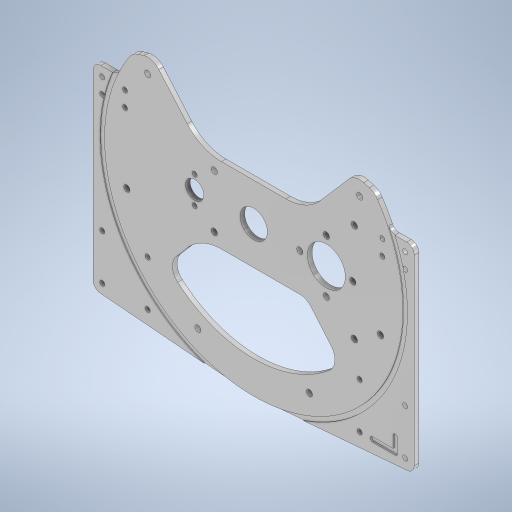
# Autodesk Inventor part: TH22_motorboard_775_v3
Saved by Autodesk Inventor 2024.1 (Build 281209000, 209)
## iProperties
Created: 2021-11-15
Part Number: TH22_motorboard_775_v3
Material: アルミニウム 6061-AHC
Document SubType Name: Modeling
Designer: 中島 青蔵
Density: 2.7 g/cm^3
Appearance: アルミニウム - ダーク
Author: 中島 青蔵
Autodesk Inventor part; units mm, degrees
ref_plane "YZ Plane" through (0, 0, 0) normal (1, 0, 0) x (0, 1, 0)
ref_plane "XZ Plane" through (0, 0, 0) normal (0, 1, 0) x (-1, 0, 0)
ref_plane "XY Plane" through (0, 0, 0) normal (0, 0, 1) x (1, 0, 0)
sketch "スケッチ1" plane through (0, 0, 0) normal (0, 0, 1) x (1, 0, 0)
  circle A0 centre (0, 0) radius 9
  line L0 (-50, 25) -> (50, 25)
  line L1 (50, 25) -> (50, -25)
  line L2 (50, -25) -> (-50, -25)
  line L3 (-50, -25) -> (-50, 25)
  line L4 (-15.8002, 25) -> (-50, 7.5852)
  line L5 (0, 0) -> (0, 25)
  line L6 (-50, 0) -> (0, 0)
  line L7 (15.8002, 25) -> (50, 7.5852)
  line L8 (20.5424, -25) -> (50, -10)
  circle A1 centre (0, 0) radius 77
  line L9 (50, 7.5852) -> (79.5557, 42.8084)
  line L10 (50, 7.5852) -> (95.9806, 7.5852) construction
  line L11 (35, 25) -> (62.1783, 57.3898)
  line L12 (35, 25) -> (77.2819, 25) construction
  line L13 (62.1783, 57.3898) -> (79.5557, 42.8084)
  line L14 (-50, 0) -> (50, 0)
  line L15 (50, -10) -> (79.5557, -42.8084)
  line L16 (35, -25) -> (62.1783, -57.3898)
  line L17 (62.1783, -57.3898) -> (79.5557, -42.8084)
  line L18 (-50, 7.5852) -> (-79.5557, 42.8084)
  line L19 (-35, 25) -> (-62.1783, 57.3898)
  line L20 (-62.1783, 57.3898) -> (-79.5557, 42.8084)
  line L21 (-35, -25) -> (-62.1783, -57.3898)
  line L22 (-50, -10) -> (-79.5557, -42.8084)
  line L23 (-62.1783, -57.3898) -> (-79.5557, -42.8084)
  line L24 (0, 0) -> (62.2943, 45.2595)
  line L25 (0, 0) -> (74.5809, -19.1491)
  line L26 (0, 0) -> (32.785, -69.6717)
  line L27 (0, 0) -> (-62.2943, 45.2595)
  line L28 (0, 0) -> (-74.5809, -19.1491)
  line L29 (0, 0) -> (-32.785, -69.6717)
  circle A2 centre (69.98, 50.8434) radius 9.5
  circle A3 centre (69.98, 50.8434) radius 2
  circle A4 centre (0, 0) radius 86.5
  circle A5 centre (83.7824, -21.5117) radius 2
  circle A6 centre (36.8299, -78.2675) radius 2
  circle A7 centre (69.98, 50.8434) radius 5
  circle A8 centre (83.7824, -21.5117) radius 5
  circle A9 centre (36.8299, -78.2675) radius 5
  circle A10 centre (-69.98, 50.8434) radius 2
  circle A11 centre (-83.7824, -21.5117) radius 2
  circle A12 centre (-36.8299, -78.2675) radius 2
  circle A13 centre (-69.98, 50.8434) radius 5
  circle A14 centre (-83.7824, -21.5117) radius 5
  circle A15 centre (-36.8299, -78.2675) radius 5
  circle A16 centre (0, 0) radius 98.5
  circle A17 centre (-69.98, 50.8434) radius 9.5
  line L30 (-74.3377, 60.3434) -> (117.0207, 60.3434)
  line L31 (-35, 25) -> (-62.8021, 57.0667)
  line L32 (35, 25) -> (62.8021, 57.0667)
  line L33 (-62.2943, 45.2595) -> (-79.6882, 57.8968)
  line L34 (-79.6882, 57.8968) -> (-72.6529, 59.9596)
  line L35 (79.6882, 57.8968) -> (72.6529, 59.9596)
  circle A18 centre (48, 0) radius 24
  circle A19 centre (-39, 0) radius 6
  circle A20 centre (-39, 9) radius 1.6
  circle A21 centre (-39, -9) radius 1.6
  circle A22 centre (0, 0) radius 24
  circle A23 centre (-39, 0) radius 15
  point P0 (50, 7.5852)
  point P1 (49.9991, -10)
  point P2 (50, -10)
  point P3 (50, 7.5852)
  point P4 (15.8002, 25)
  point P5 (50.0002, -9.8901)
  point P6 (-50.0002, -10)
  point P7 (62.2943, 45.2595)
  point P8 (57.2394, 51.5039)
  point P9 (70.1939, 31.6514)
  point P10 (69.9626, -32.1595)
  point P11 (57.2394, -51.5039)
  point P12 (-57.2394, -51.5039)
  point P13 (-69.9626, -32.1595)
  point P14 (-70.1939, 31.6514)
  point P15 (-57.2394, 51.5039)
  point P16 (-77.6656, 56.4274)
  point P17 (77.6656, 56.4274)
  point P18 (-62.7025, 56.9499)
  point P19 (62.7025, 56.9499)
  point P20 (-62.7016, 56.9507)
  point P21 (62.7016, 56.9507)
  point P22 (53.3257, -13.6917)
  point P23 (46.2951, -11.8866)
  point P24 (11.7641, -25)
  dimension "d78" = 197
  dimension "d0" = 18
  dimension "d7" = 50
  dimension "d27" = 100
  dimension "d43" = 154
  dimension "d44" = 50
  dimension "d45" = 50
  dimension "d58" = 25
  dimension "d59" = 15
  dimension "d63" = 15
  dimension "d67" = 15
  dimension "d68" = 54
  dimension "d69" = 50.4
  dimension "d70" = 50.4
  dimension "d71" = 19
  dimension "d72" = 4
  dimension "d73" = 4
  dimension "d74" = 4
  dimension "d75" = 10
  dimension "d76" = 10
  dimension "d77" = 10
  dimension "d118" = 48
  dimension "d119" = 48
  dimension "d172" = 12
  dimension "d173" = 3.2
  dimension "d174" = 3.2
  dimension "d175" = 9
  dimension "d176" = 9
  dimension "d177" = 48
  dimension "d178" = 30
  dimension "d179" = 0
  dimension "d180" = 0
  constraints: 72 end point, 26 symmetric about line, 23 centre point, 14 coincident, 9 point on line, 8 point on circle, 6 tangent, 3 midpoint, 3 perpendicular, 2 equal length, 2 horizontal, 1 collinear, 1 parallel, 1 vertical, 10 other
  measures "d0" diameter of A0
  measures "d7" distance of L0.end L1.end
  measures "d27" distance of L0.start L0.end
  measures "d43" diameter of A1
  measures "d44" angle of L10 L9
  measures "d45" angle of L12 L11
  measures "d58" distance from line of point (0, 0) L2
  measures "d59" distance from line of L2 L8.end
  measures "d63" distance of L0.end L11.start
  measures "d67" distance of L2.end point (-50, -10)
  measures "d68" angle of L5 L24
  measures "d69" angle of L24 L25
  measures "d70" angle of L25 L26
  measures "d71" diameter of A2
  measures "d72" diameter of A3
  measures "d73" diameter of A5
  measures "d74" diameter of A6
  measures "d75" diameter of A7
  measures "d76" diameter of A8
  measures "d77" diameter of A9
  measures "d118" distance of point (0, 0) point (48, 0)
  measures "d119" diameter of A18
  measures "d172" diameter of A19
  measures "d173" diameter of A20
  measures "d174" diameter of A21
  measures "d175" distance of A19.centre A20.centre
  measures "d176" distance of A21.centre A19.centre
  measures "d177" diameter of A22
  measures "d178" diameter of A23
  measures "d179" horizontal distance of A19.centre A20.centre
  measures "d180" horizontal distance of A19.centre A21.centre
extrude "押し出し1" add sketch "スケッチ1" along normal blind 3 contours L14 A22 L25 A0 | A0 L24 A22 L14 | A0 L5 A22 L24 | L25 A22 L26 A0 | A18 L7 L1 L14 | A22 L24 L7 A18 | L14 L1 L8 L25 A18 | A18 L25 A22 | A0 L27 A22 L5 | A22 L5 L0 L7 L24 | L26 A22 L29 A0 | L25 A18 L8 L2 L26 A22 | L6 A22 L27 A0 | A0 L28 A22 L6 | A0 L29 A22 L28 | L1 L9 A18 L25 L15 | A18 L1 L7 | L7 L24 L0 L1 A18 | L25 L8 A18 | A22 L27 L4 L0 L5 | L7 L0 L24 | L26 L2 L29 A22 | A23 L28 A21 L3 L6 A19 | A23 L4 L27 A22 | L6 A19 L3 L4 A23 | A22 L28 A23 | A22 L29 L2 L3 L28 A23 | L1 A18 L9 | L15 L25 L1 | L1 L25 L8 | L1 L0 L32 L24 A1 L9 A18 | L25 L1 A18 L8 | A18 L1 L2 L8 | A23 L3 L0 L27 L4 | L4 L3 A23 | A23 L28 A21 | L27 L0 L4 | L9 A1 L25 A18 | L25 L15 A18 L1 | L25 A18 L15 | A18 L15 A1 L16 L2 L1 | A1 L16 L17 A4 A9 A15 L23 L21 | L18 A23 L3 | L3 L22 A23 L18 | A23 L18 A1 L27 L31 L0 L3 | L28 L3 A23 | L21 A1 L22 L28 L3 L2 | L9 A4 A8 L15 A1 | A1 A2 A4 L9 | A18 L25 A1 L15 | L32 A1 L24 | A1 L15 A4 L17 L16 | A23 L22 L28 A1 L18 | L28 L22 A23 L3 | A23 L22 L3 | L21 L23 A4 L22 A1 | A1 L32 A2 | A2 L13 A7 A4 | A4 A2 L13 L9 | L9 L13 A2 L35 A16 L33 A17 L20 L18 A4 A14 L22 L23 A15 A9 L17 L15 A8 | L18 A4 A17 A1 | A1 L22 A4 A14 L18 | L22 A1 L28 | L27 A1 L31 | A2 A4 A7 L13 | A4 A7 L13 A2 | L15 L17 A4 | A17 L31 A1 | L33 A13 L20 A17 | A17 A4 A13 L33 | L18 L20 A17 A4 | A4 L23 L22 | A7 A4 A3 L13 | L13 A3 A4 A7 | L13 A7 A4 A2 | A4 A3 L13 A7 | A8 A4 A5 | A4 A5 A8 | A9 A4 A6 | A4 A6 A9 | A17 L20 A13 A4 | L33 A10 L20 A13 | A13 A4 A10 L33 | A14 A4 A11 | A4 A11 A14 | L20 A13 A4 A17 | A15 A4 A12 | A4 A12 A15 | A7 L13 A3 A4 | A4 A13 L33 A17 | A13 L20 A10 A4 | A17 L33 A13 L20 | L20 A10 A4 A13 | A4 A10 L33 A13 | A17 L33 L34 | A13 L33 A10 L20
fillet "フィレット2" radius 30 3 edges at (35, 25, 1.5) (-35, -25, 1.5) (-35, 25, 1.5)
fillet "フィレット5" radius 10 5 edges at (-79.6882, 57.8968, 1.5) (79.6882, 57.8968, 1.5) (-57.2394, -51.5039, 1.5) (35, -25, 1.5) (57.2394, -51.5039, 1.5)
sketch "スケッチ6" plane through (0, 0, 3) normal (0, 0, 1) x (1, 0, 0)
  point P0 (0, 0)
  point P1 (48, 0)
  point P2 (48, 17.5)
  point P3 (30.5, 0)
  point P4 (48, -17.5)
  point P5 (65.5, 0)
  dimension "d81" = 48
  dimension "d82" = 17.5
  dimension "d85" = 360
  constraints: 5 other
  measures "d81" distance of point (0, 0) point (48, 0)
  measures "d82" distance of point (48, 0) point (48, 17.5)
hole "穴4" at (48, 0, 3) direction (0, 0, -1) diameter 25 depth 8 tip angle 118
hole "穴5" at (48, 17.5, 3) at (30.5, 0, 3) at (48, -17.5, 3) at (65.5, 0, 3) direction (0, 0, -1) diameter 4 depth 8 tip angle 118
sketch "スケッチ7" plane through (0, 0, 3) normal (0, 0, 1) x (1, 0, 0)
  line L0 (21.3047, 25) -> (-21.3047, 25) projected
  line L1 (-21.0108, -25) -> (30.3369, -25) projected
  circle A0 centre (48, 0) radius 12.5 projected
  point P0 (0, 0)
  point P1 (-26, 17.5)
  point P2 (-26, -17.5)
  point P3 (66.5, -32.5)
  point P4 (66.5, 32.5)
  point P5 (21.0108, -25)
  point P6 (11.7641, -25)
  point P7 (5.4179, -25)
  point P8 (25.7007, -25)
  point P9 (-35, -25)
  point P10 (35, -25)
  point P11 (-30.3369, -25)
  dimension "d101" = 26
  dimension "d102" = 7.5
  dimension "d103" = 26
  dimension "d104" = 7.5
  dimension "d105" = 18.5
  dimension "d106" = 18.5
  dimension "d116" = 7.5
  dimension "d117" = 7.5
  constraints: 1 other
  measures "d101" horizontal distance of point (0, 0) point (-26, 17.5)
  measures "d102" distance from line of L0 point (-26, 17.5)
  measures "d103" horizontal distance of point (-26, -17.5) point (0, 0)
  measures "d105" horizontal distance of A0.centre point (66.5, 32.5)
  measures "d106" horizontal distance of A0.centre point (66.5, -32.5)
  measures "d116" distance from line of L0 point (66.5, 32.5)
hole "穴6" at (-26, 17.5, 3) at (-26, -17.5, 3) at (66.5, -32.5, 3) at (66.5, 32.5, 3) direction (0, 0, -1) diameter 4 depth 8 tip angle 118
sketch "スケッチ8" plane through (0, 0, 3) normal (0, 0, 1) x (1, 0, 0)
  arc A0 (-81.8095, 54.8585) -> (81.8095, 54.8585) centre (0, 0) ccw projected
  circle A1 centre (83.7824, -21.5117) radius 2 projected
  line L0 (89.9517, 40.1366) -> (106, 40.1366)
  line L1 (106, 40.1366) -> (106, -89.8634)
  line L2 (106, -89.8634) -> (8.3243, -98.1476)
  line L3 (0, 0) -> (0, -98.5)
  circle A2 centre (100, 34.1366) radius 1.6
  circle A3 centre (100, -83.8634) radius 1.6
  line L4 (-89.9517, 40.1366) -> (-106, 40.1366)
  line L5 (-106, 40.1366) -> (-106, -89.8634)
  line L6 (-106, -89.8634) -> (-8.3243, -98.1476)
  circle A4 centre (-100, 34.1366) radius 1.6
  circle A5 centre (-100, -83.8634) radius 1.6
  point P0 (-8.3243, -98.1476)
  point P1 (-89.9517, 40.1366)
  dimension "d132" = 130
  dimension "d133" = 3.2
  dimension "d134" = 3.2
  dimension "d135" = 6
  dimension "d136" = 6
  dimension "d137" = 6
  dimension "d138" = 6
  dimension "d155" = 85.152
  dimension "d156" = 100
  constraints: 14 end point, 6 symmetric about line, 4 centre point, 3 point on circle, 1 horizontal, 1 tangent, 1 vertical, 2 other
  measures "d132" distance of L0.end L1.end
  measures "d133" diameter of A2
  measures "d134" diameter of A3
  measures "d135" distance from line of L0 A2.centre
  measures "d136" distance from line of L1 A2.centre
  measures "d137" distance from line of L1 A3.centre
  measures "d138" horizontal distance of L1.end A3.centre
  measures "d155" angle of L3 L2
  measures "d156" horizontal distance of point (0, 0) A2.centre
extrude "押し出し2" add sketch "スケッチ8" against normal blind 3 contours A0 L6 L5 L4 | A0 L0 L1 L2
fillet "フィレット8" radius 5 6 edges at (106, 40.1366, 1.5) (106, -89.8634, 1.5) (-106, -89.8634, 1.5) (-106, 40.1366, 1.5) (-89.9517, 40.1366, 1.5) (89.9517, 40.1366, 1.5)
sketch "スケッチ9" plane through (0, 0, 3) normal (0, 0, 1) x (1, 0, 0)
  arc A0 (-81.8095, 54.8585) -> (81.8095, 54.8585) centre (0, 0) ccw projected
  circle A1 centre (0, 0) radius 101.5
  arc A2 (88.6399, 42.9561) -> (93.1393, 40.1366) centre (93.1393, 45.1366) ccw projected
  line L0 (8.3243, -98.1476) -> (101.4226, -90.2516) projected
  line L1 (-101.4226, -90.2516) -> (-8.3243, -98.1476) projected
  arc A3 (-93.1393, 40.1366) -> (-88.6399, 42.9561) centre (-93.1393, 45.1366) ccw projected
  circle A4 centre (78.5, -83.8634) radius 1.5
  circle A5 centre (93.5, -74.8634) radius 1.5
  circle A6 centre (100, -83.8634) radius 1.6 projected
  circle A7 centre (93.5, -83.8634) radius 1.5
  line L2 (78.5, -82.3634) -> (93.5, -82.3634)
  line L3 (93.5, -85.3634) -> (78.5, -85.3634)
  line L4 (92, -74.8634) -> (92, -83.8634)
  line L5 (95, -83.8634) -> (95, -74.8634)
  line L6 (101, 40.1366) -> (93.1393, 40.1366) projected
  line L7 (-93.1393, 40.1366) -> (-101, 40.1366) projected
  point P0 (-96.9226, 30.1373)
  point P1 (-32.7315, -96.0776)
  point P2 (32.7315, -96.0776)
  point P3 (96.9226, 30.1373)
  point P4 (92, -82.3634)
  point P5 (-93.2272, 40.1366)
  point P6 (93.2272, 40.1366)
  dimension "d142" = 203
  dimension "d146" = 3
  dimension "d147" = 3
  dimension "d148" = 0
  dimension "d149" = 3
  dimension "d150" = 6.5
  dimension "d151" = 15
  dimension "d152" = 9
  constraints: 8 end point, 8 point on circle, 4 centre point, 2 horizontal, 2 vertical, 1 coincident
  measures "d142" diameter of A1
  measures "d146" diameter of A4
  measures "d147" diameter of A5
  measures "d148" vertical distance of A6.centre A4.centre
  measures "d149" diameter of A7
  measures "d150" distance of A6.centre A7.centre
  measures "d151" distance of A7.centre A4.centre
  measures "d152" distance of A7.centre A5.centre
extrude "押し出し3" cut sketch "スケッチ9" against normal blind 0.5 contours A0 L1 A1 L7 A3 | A0 A2 L6 A1 L0
extrude "押し出し4" cut sketch "スケッチ9" against normal blind 1 contours A4 | A4 L2 L4 A7 L3 | L4 A5 L5 A7 L2 | L2 A7 L4 | A7 | A5
sketch "スケッチ10" plane through (0, 0, 3) normal (0, 0, 1) x (1, 0, 0)
  circle A0 centre (-100, 34.1366) radius 1.6 projected
  circle A1 centre (-100, -83.8634) radius 1.6 projected
  line L0 (0, 25) -> (0, -25)
  line L1 (21.3047, 25) -> (-21.3047, 25) projected
  line L2 (-21.0108, -25) -> (30.3369, -25) projected
  point P0 (0, 0)
  point P1 (-100, 24.1366)
  point P2 (-85, 24.1366)
  point P3 (-85, 34.1366)
  point P4 (-100, -53.8634)
  point P5 (-70, -53.8634)
  point P6 (-70, -83.8634)
  point P7 (15.4822, -25)
  point P8 (100, 24.1366)
  point P9 (85, 24.1366)
  point P10 (85, 34.1366)
  point P11 (100, -53.8634)
  point P12 (70, -53.8634)
  point P13 (70, -83.8634)
  point P14 (-35, -25)
  point P15 (35, -25)
  point P16 (-30.3369, -25)
  dimension "d157" = 10
  dimension "d158" = 15
  dimension "d159" = 10
  dimension "d160" = 15
  dimension "d161" = 30
  dimension "d162" = 30
  dimension "d163" = 30
  dimension "d164" = 30
  constraints: 6 symmetric about line, 2 end point, 1 midpoint, 1 point on line, 1 vertical
  measures "d157" distance of point (-100, 24.137) A0.centre
  measures "d158" distance of point (-85, 34.137) A0.centre
  measures "d159" vertical distance of A0.centre point (-85, 24.137)
  measures "d160" horizontal distance of point (-85, 24.137) A0.centre
  measures "d161" distance of A1.centre point (-100, -53.863)
  measures "d162" distance of A1.centre point (-70, -83.863)
  measures "d163" horizontal distance of A1.centre point (-70, -53.863)
  measures "d164" horizontal distance of A1.centre point (-70, -53.863)
hole "穴7" at (-100, 24.1366, 3) at (-85, 24.1366, 3) at (-85, 34.1366, 3) at (-100, -53.8634, 3) at (-70, -53.8634, 3) at (-70, -83.8634, 3) at (85, 34.1366, 3) at (100, 24.1366, 3) at (85, 24.1366, 3) at (100, -53.8634, 3) at (70, -53.8634, 3) at (70, -83.8634, 3) direction (0, 0, -1) diameter 3.2 end through all
